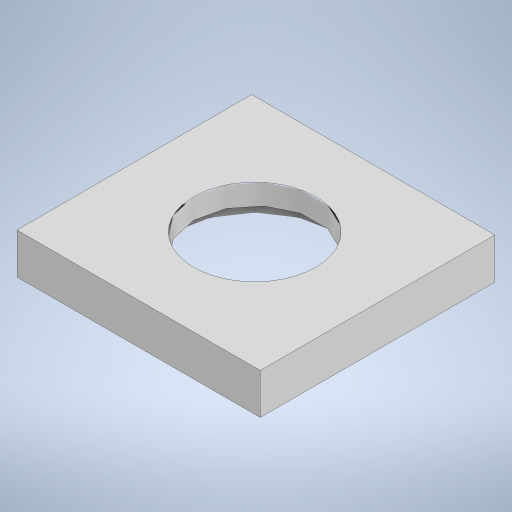
# Autodesk Inventor part: Button_slot
Saved by Autodesk Inventor 2023 (Build 270158000, 158)
## iProperties
Created: 2022-11-29
Part Number: Button_slot
Material: Generic
Document SubType Name: Modeling
Designer: spfow
Density: 1 g/cm^3
Appearance: Default
Author: spfow
Autodesk Inventor part; units mm, degrees
note: some values were not read from the file. Chosen so that the rebuilt part matches the saved one: offset side.
ref_plane "YZ Plane" through (0, 0, 0) normal (1, 0, 0) x (0, 1, 0)
ref_plane "XZ Plane" through (0, 0, 0) normal (0, 1, 0) x (-1, 0, 0)
ref_plane "XY Plane" through (0, 0, 0) normal (0, 0, 1) x (1, 0, 0)
sketch "Sketch1" plane through (0, 0, 0) normal (0, 1, 0) x (-1, 0, 0)
  line L0 (0, 0) -> (177.8, 0)
  line L1 (177.8, 0) -> (177.8, -114.3)
  line L2 (177.8, -114.3) -> (0, -114.3)
  line L3 (0, -114.3) -> (0, 0)
  dimension "d0" = 177.8
  dimension "d1" = 114.3
  constraints: 8 end point, 2 parallel, 1 horizontal, 1 perpendicular
  measures "d0" distance of L1.end L2.end
  measures "d1" distance of L0.end L1.end
extrude "Extrusion1" add sketch "Sketch1" along normal blind 38.1
sketch "Sketch2" plane through (0, 0, 0) normal (0, -1, 0) x (1, 0, 0)
  line L0 (-177.8, -114.3) -> (-177.8, 0) projected
  line L1 (0, 0) -> (-177.8, 0)
  line L2 (-177.8, 0) -> (-177.8, -114.3)
  line L3 (-177.8, -114.3) -> (0, -114.3)
  line L4 (0, -114.3) -> (0, 0)
  line L5 (-5.08, -5.08) -> (-172.72, -5.08)
  line L6 (-172.72, -5.08) -> (-172.72, -109.22)
  line L7 (-172.72, -109.22) -> (-5.08, -109.22)
  line L8 (-5.08, -109.22) -> (-5.08, -5.08)
  dimension "d4" = 5.08
  constraints: 16 end point, 4 parallel, 2 perpendicular, 1 horizontal, 3 other
  measures "d4" distance between parallel lines of L4 L8
extrude "Extrusion2" cut sketch "Sketch2" against normal blind 35.56 contours L8 L7 L6 L5
fillet "Fillet1" radius 3.175 4 edges at (-177.8, 38.1, -57.15) (-88.9, 38.1, 0) (-88.9, 38.1, -114.3) (0, 38.1, -57.15)
sketch "Sketch3" plane through (0, 38.1, 0) normal (0, 1, 0) x (1, 0, 0)
  line L0 (-177.8, 114.3) -> (-171.45, 114.3)
  line L1 (-171.45, 114.3) -> (-171.45, 0)
  line L2 (-171.45, 0) -> (-177.8, 0)
  line L3 (-177.8, 0) -> (-177.8, 114.3)
  line L4 (0, 114.3) -> (-177.8, 114.3) projected
  line L5 (-177.8, 114.3) -> (0, 114.3)
  line L6 (0, 114.3) -> (0, 107.95)
  line L7 (0, 107.95) -> (-177.8, 107.95)
  line L8 (-177.8, 107.95) -> (-177.8, 114.3)
  line L9 (-158.75, 100.4887) -> (-100.6475, 100.4887)
  line L10 (-100.6475, 100.4887) -> (-100.6475, 13.8112)
  line L11 (-100.6475, 13.8112) -> (-158.75, 13.8112)
  line L12 (-158.75, 13.8112) -> (-158.75, 100.4887)
  point P0 (0, 0)
  dimension "d8" = 6.35
  dimension "d9" = 6.35
  dimension "d10" = 58.1025
  dimension "d11" = 86.6775
  dimension "d12" = 13.8112
  dimension "d13" = 19.05
  constraints: 24 end point, 6 parallel, 3 horizontal, 3 perpendicular
  measures "d8" distance of L1.end L2.end
  measures "d9" distance of L5.end L6.end
  measures "d10" distance of L9.start L9.end
  measures "d11" distance of L9.end L10.end
  measures "d12" distance between parallel lines of L4 L9
  measures "d13" distance between parallel lines of L3 L12
extrude "Extrusion3" cut sketch "Sketch3" against normal blind 35.56 contours L9 L10 L11 L12
sketch "Sketch4" plane through (0, 38.1, 0) normal (0, 1, 0) x (1, 0, 0)
  line L0 (-94.2975, 17.78) -> (-81.2088, 17.78)
  line L1 (-91.7575, 20.32) -> (-91.7575, 26.67)
  line L2 (-91.7575, 26.67) -> (-94.2975, 26.67)
  line L3 (-94.2975, 26.67) -> (-94.2975, 17.78)
  line L4 (-94.2975, 17.78) -> (-78.6765, 17.78)
  line L5 (-78.6765, 17.78) -> (-78.6765, 20.32)
  line L6 (-94.2975, 24.2647) -> (-94.2975, 17.78)
  line L7 (-85.6615, 20.32) -> (-85.6615, 24.13)
  line L8 (-85.6615, 24.13) -> (-88.2015, 24.13)
  line L9 (-88.2015, 24.13) -> (-88.2015, 20.32)
  line L10 (-78.6765, 20.32) -> (-85.6615, 20.32)
  line L11 (-88.2015, 20.32) -> (-91.7575, 20.32)
  line L12 (-100.6475, 100.4887) -> (-100.6475, 13.8112) projected
  line L13 (-177.8, 0) -> (0, 0) projected
  line L14 (-94.2975, 27.94) -> (-78.6765, 27.94)
  line L15 (-78.6765, 27.94) -> (-78.6765, 30.7699)
  line L16 (-81.2165, 30.48) -> (-94.2975, 30.48)
  line L17 (-94.2975, 30.48) -> (-94.2975, 27.94)
  line L18 (-83.0828, 27.94) -> (-78.6765, 27.94)
  line L19 (-78.6765, 27.94) -> (-78.6765, 36.83)
  line L20 (-78.6765, 36.83) -> (-81.2165, 36.83)
  line L21 (-81.2165, 36.83) -> (-81.2165, 30.48)
  ellipse E0 centre (-86.487, 41.91) end of major axis (-94.2975, 41.91) minor radius 5.334
  ellipse E1 centre (-86.487, 53.34) end of major axis (-94.2975, 53.34) minor radius 5.334
  line L22 (-94.2975, 60.96) -> (-78.6765, 60.96)
  line L23 (-78.6765, 60.96) -> (-78.6765, 63.754)
  line L24 (-94.2975, 63.754) -> (-94.2975, 60.96)
  ellipse E2 centre (-86.487, 63.754) end of major axis (-94.2975, 63.754) minor radius 7.62 (-78.6765, 63.754) -> (-94.2975, 63.754) ccw
  line L25 (-91.7575, 63.754) -> (-91.7575, 63.5)
  line L26 (-91.7575, 63.5) -> (-81.2165, 63.5)
  line L27 (-81.2165, 63.5) -> (-81.2165, 63.754)
  line L28 (-94.2975, 82.55) -> (-78.6765, 82.55)
  line L29 (-78.6765, 82.55) -> (-78.6765, 80.01)
  line L30 (-78.6765, 80.01) -> (-94.2975, 80.01)
  line L31 (-94.2975, 80.01) -> (-94.2975, 82.55)
  line L32 (-91.7575, 89.535) -> (-78.6765, 89.535)
  line L33 (-78.6765, 89.535) -> (-78.6765, 92.075)
  line L34 (-78.6765, 92.075) -> (-91.7575, 92.075)
  line L35 (-94.2975, 94.8241) -> (-94.2975, 91.9305)
  line L36 (-94.2975, 85.09) -> (-91.7575, 85.09)
  line L37 (-91.7575, 96.52) -> (-94.2975, 96.52)
  line L38 (-94.2975, 96.52) -> (-94.2975, 85.09)
  line L39 (-91.7575, 85.09) -> (-91.7575, 89.535)
  line L40 (-91.7575, 92.075) -> (-91.7575, 96.52)
  spline S0 degree 5 poles (-91.7575, 41.91) (-91.7584, 41.6813) (-91.6944, 41.4527) (-91.5885, 41.2473) (-91.2042, 40.6846) (-90.6636, 40.2564) (-90.282, 40.0177) (-89.3306, 39.5478) (-88.3046, 39.2718) (-87.7026, 39.1679) (-86.487, 39.0641) (-85.2714, 39.1679) (-84.6694, 39.2718) (-83.6435, 39.5478) (-82.692, 40.0176) (-82.3107, 40.2563) (-81.7696, 40.6845) (-81.3858, 41.2473) (-81.2787, 41.4526) (-81.1539, 41.91) (-81.2787, 42.3674) (-81.3858, 42.5727) (-81.7696, 43.1355) (-82.3107, 43.5637) (-82.692, 43.8024) (-83.6435, 44.2722) (-84.6694, 44.5482) (-85.2714, 44.6521) (-86.487, 44.7559) (-87.7026, 44.6521) (-88.3046, 44.5482) (-89.3306, 44.2722) (-90.282, 43.8023) (-90.6636, 43.5636) (-91.2042, 43.1354) (-91.5885, 42.5727) (-91.6944, 42.3673) (-91.7584, 42.1387) (-91.7575, 41.91) knots 0 0 0 0 0 0 0.044471 0.044471 0.044471 0.131758 0.131758 0.131758 0.25 0.25 0.25 0.36824 0.36824 0.36824 0.455522 0.455522 0.455522 0.5 0.5 0.5 0.544478 0.544478 0.544478 0.63176 0.63176 0.63176 0.75 0.75 0.75 0.868242 0.868242 0.868242 0.955529 0.955529 0.955529 1 1 1 1 1 1
  spline S1 degree 5 poles (-91.7575, 53.34) (-91.7584, 53.1113) (-91.6944, 52.8827) (-91.5885, 52.6773) (-91.2042, 52.1146) (-90.6636, 51.6864) (-90.282, 51.4477) (-89.3306, 50.9778) (-88.3046, 50.7018) (-87.7026, 50.5979) (-86.487, 50.4941) (-85.2714, 50.5979) (-84.6694, 50.7018) (-83.6435, 50.9778) (-82.692, 51.4476) (-82.3107, 51.6863) (-81.7696, 52.1145) (-81.3858, 52.6773) (-81.2787, 52.8826) (-81.1539, 53.34) (-81.2787, 53.7974) (-81.3858, 54.0027) (-81.7696, 54.5655) (-82.3107, 54.9937) (-82.692, 55.2324) (-83.6435, 55.7022) (-84.6694, 55.9782) (-85.2714, 56.0821) (-86.487, 56.1859) (-87.7026, 56.0821) (-88.3046, 55.9782) (-89.3306, 55.7022) (-90.282, 55.2323) (-90.6636, 54.9936) (-91.2042, 54.5654) (-91.5885, 54.0027) (-91.6944, 53.7973) (-91.7584, 53.5687) (-91.7575, 53.34) knots 0 0 0 0 0 0 0.044471 0.044471 0.044471 0.131758 0.131758 0.131758 0.25 0.25 0.25 0.36824 0.36824 0.36824 0.455522 0.455522 0.455522 0.5 0.5 0.5 0.544478 0.544478 0.544478 0.63176 0.63176 0.63176 0.75 0.75 0.75 0.868242 0.868242 0.868242 0.955529 0.955529 0.955529 1 1 1 1 1 1
  spline S2 degree 5 poles (-81.2165, 63.754) (-81.2166, 64.309) (-81.2953, 64.8639) (-81.4525, 65.404) (-82.1282, 66.8995) (-83.3585, 68.0474) (-84.3453, 68.5716) (-86.487, 69.0964) (-88.6287, 68.5716) (-89.6155, 68.0474) (-90.8458, 66.8995) (-91.5215, 65.404) (-91.6787, 64.8639) (-91.7574, 64.309) (-91.7575, 63.754) knots 0 0 0 0 0 0 0.170659 0.170659 0.170659 0.5 0.5 0.5 0.829341 0.829341 0.829341 1 1 1 1 1 1
  point P0 (-94.2975, 93.3773)
  point P1 (-88.9, 0)
  point P2 (-93.0275, 85.09)
  dimension "d32" = 5.334
  dimension "d33" = 7.8105
  dimension "d36" = 7.8105
  dimension "d37" = 5.334
  dimension "d42" = 7.62
  dimension "d43" = 2.54
  dimension "d16" = 2.54
  dimension "d17" = 3.556
  dimension "d18" = 2.54
  dimension "d19" = 6.985
  dimension "d20" = 8.89
  dimension "d21" = 6.35
  dimension "d22" = 3.81
  dimension "d23" = 3.81
  dimension "d24" = 6.35
  dimension "d25" = 17.78
  dimension "d26" = 2.54
  dimension "d27" = 2.54
  dimension "d28" = 6.35
  dimension "d29" = 15.621
  dimension "d30" = 6.35
  dimension "d31" = 27.94
  dimension "d34" = 14.1605
  dimension "d35" = 41.91
  dimension "d38" = 14.1605
  dimension "d39" = 53.34
  dimension "d40" = 2.54
  dimension "d41" = 2.54
  dimension "d44" = 6.35
  dimension "d45" = 15.621
  dimension "d46" = 60.96
  dimension "d47" = 2.794
  dimension "d48" = 63.754
  dimension "d49" = 14.1605
  dimension "d50" = 2.54
  dimension "d51" = 15.621
  dimension "d52" = 4.445
  dimension "d53" = 4.445
  dimension "d54" = 2.54
  dimension "d55" = 2.54
  dimension "d56" = 6.35
  dimension "d57" = 80.01
  dimension "d58" = 2.54
  dimension "d59" = 13.081
  dimension "d62" = 3.9688
  dimension "d63" = 3.9688
  constraints: 78 end point, 20 parallel, 10 perpendicular, 8 horizontal, 5 point on line, 3 midpoint, 13 other
  measures "d16" distance of L1.end L2.end
  measures "d17" distance of L9.end L1.start
  measures "d18" distance of L7.end L8.end
  measures "d19" distance of L5.end L7.start
  measures "d20" distance of L2.end L0.start
  measures "d21" distance of L1.start L1.end
  measures "d22" distance of L8.end L9.end
  measures "d23" distance of L7.start L7.end
  measures "d24" distance between parallel lines of L12 L3
  measures "d25" distance between parallel lines of L13 L0
  measures "d26" distance of L16.end L14.start
  measures "d27" distance of L19.end L20.end
  measures "d28" distance of L20.end L16.start
  measures "d29" distance of L14.start L14.end
  measures "d30" distance between parallel lines of L12 L17
  measures "d31" distance between parallel lines of L13 L14
  measures "d34" distance from line of L12 point (-86.487, 41.91)
  measures "d35" distance from line of L13 point (-86.487, 41.91)
  measures "d38" distance from line of L12 point (-86.487, 53.34)
  measures "d39" distance from line of L13 point (-86.487, 53.34)
  measures "d44" distance between parallel lines of L12 L24
  measures "d45" distance of L22.start L22.end
  measures "d46" distance between parallel lines of L13 L22
  measures "d47" distance of L24.start L22.start
  measures "d48" distance from line of L13 point (-86.487, 63.754)
  measures "d49" distance from line of L12 point (-86.487, 63.754)
  measures "d50" distance of L30.end L28.start
  measures "d51" distance of L29.end L30.end
  measures "d52" distance of L36.end L32.start
  measures "d53" distance of L34.end L37.start
  measures "d54" distance between parallel lines of L32 L34
  measures "d55" distance between parallel lines of L40 L38
  measures "d56" distance from line of L12 point (-94.298, 93.377)
  measures "d57" distance from line of point (-88.9, 0) L30
  measures "d58" distance from line of L28 point (-93.028, 85.09)
  measures "d59" distance of L32.start L32.end
  measures "d62" distance from line of L12.start L37
  measures "d63" distance from line of L12.end L0
extrude "Extrusion4" cut sketch "Sketch4" against normal blind 1.27
sketch "Sketch5" plane through (0, 38.1, 0) normal (0, 1, 0) x (1, 0, 0)
  line L0 (-43.4975, 22.6219) -> (-37.9413, 22.6219)
  line L1 (-37.9413, 22.6219) -> (-37.9413, 28.1781)
  line L2 (-37.9413, 28.1781) -> (-43.4975, 28.1781)
  line L3 (-43.4975, 28.1781) -> (-43.4975, 22.6219)
  line L4 (-43.4975, 38.4969) -> (-37.9413, 38.4969)
  line L5 (-37.9413, 38.4969) -> (-37.9413, 44.0531)
  line L6 (-37.9413, 44.0531) -> (-43.4975, 44.0531)
  line L7 (-43.4975, 44.0531) -> (-43.4975, 38.4969)
  line L8 (-43.4975, 54.3719) -> (-37.9413, 54.3719)
  line L9 (-37.9413, 54.3719) -> (-37.9413, 59.9281)
  line L10 (-37.9413, 59.9281) -> (-43.4975, 59.9281)
  line L11 (-43.4975, 59.9281) -> (-43.4975, 54.3719)
  line L12 (-43.4975, 70.2469) -> (-37.9413, 70.2469)
  line L13 (-37.9413, 70.2469) -> (-37.9413, 75.8031)
  line L14 (-37.9413, 75.8031) -> (-43.4975, 75.8031)
  line L15 (-43.4975, 75.8031) -> (-43.4975, 70.2469)
  line L16 (-43.4975, 86.1219) -> (-37.9413, 86.1219)
  line L17 (-37.9413, 86.1219) -> (-37.9413, 91.6781)
  line L18 (-37.9413, 91.6781) -> (-43.4975, 91.6781)
  line L19 (-43.4975, 91.6781) -> (-43.4975, 86.1219)
  line L20 (0, 114.3) -> (-177.8, 114.3) projected
  line L21 (-177.8, 0) -> (0, 0) projected
  line L22 (-100.6475, 100.4887) -> (-100.6475, 13.8112) projected
  circle A0 centre (-21.9075, 25.4) radius 3.81
  circle A1 centre (-21.9075, 41.275) radius 3.81
  circle A2 centre (-21.9075, 57.15) radius 3.81
  circle A3 centre (-21.9075, 73.025) radius 3.81
  circle A4 centre (-21.9075, 88.9) radius 3.81
  point P0 (-43.4975, 73.025)
  dimension "d64" = 5.5563
  dimension "d65" = 5.5563
  dimension "d66" = 5.5563
  dimension "d67" = 5.5563
  dimension "d68" = 5.5563
  dimension "d69" = 5.5563
  dimension "d70" = 15.875
  dimension "d71" = 15.875
  dimension "d72" = 15.875
  dimension "d73" = 15.875
  dimension "d74" = 22.6219
  dimension "d76" = 57.15
  dimension "d77" = 7.62
  dimension "d78" = 7.62
  dimension "d79" = 7.62
  dimension "d80" = 7.62
  dimension "d81" = 7.62
  dimension "d82" = 15.875
  dimension "d83" = 15.875
  dimension "d84" = 15.875
  dimension "d85" = 15.875
  dimension "d86" = 25.4
  dimension "d87" = 78.74
  dimension "d88" = 78.74
  dimension "d89" = 78.74
  dimension "d90" = 78.74
  dimension "d91" = 78.74
  constraints: 40 end point, 10 parallel, 8 point on line, 5 centre point, 5 horizontal, 5 perpendicular, 1 midpoint
  measures "d64" distance of L2.end L0.start
  measures "d65" distance of L6.end L4.start
  measures "d66" distance of L10.end L8.start
  measures "d67" distance of L14.end L12.start
  measures "d68" distance of L18.end L16.start
  measures "d69" distance of L17.end L18.end
  measures "d70" distance of L5.end L1.end
  measures "d71" distance of L9.end L5.end
  measures "d72" distance of L13.end L9.end
  measures "d73" distance of L17.end L13.end
  measures "d74" distance between parallel lines of L20 L18
  measures "d76" distance from line of point (-43.498, 73.025) L22
  measures "d77" diameter of A0
  measures "d78" diameter of A1
  measures "d79" diameter of A2
  measures "d80" diameter of A3
  measures "d81" diameter of A4
  measures "d82" distance of A1.centre A0.centre
  measures "d83" distance of A2.centre A1.centre
  measures "d84" distance of A3.centre A2.centre
  measures "d85" distance of A4.centre A3.centre
  measures "d86" distance from line of L20 A4.centre
  measures "d87" distance from line of L22 A2.centre
  measures "d88" distance from line of L22 A3.centre
  measures "d89" distance from line of L22 A4.centre
  measures "d90" distance from line of L22 A1.centre
  measures "d91" distance from line of L22 A0.centre
extrude "Extrusion5" cut sketch "Sketch5" against normal blind 25.4
sketch "Sketch6" plane through (0, 35.56, 0) normal (0, -1, 0) x (1, 0, 0)
  circle A0 centre (-21.9075, -88.9) radius 3.81 projected
  circle A1 centre (-21.9075, -88.9) radius 5.08
  circle A2 centre (-21.9075, -73.025) radius 3.81 projected
  circle A3 centre (-21.9075, -73.025) radius 5.08
  circle A4 centre (-21.9075, -57.15) radius 3.81 projected
  circle A5 centre (-21.9075, -57.15) radius 5.08
  circle A6 centre (-21.9075, -41.275) radius 3.81 projected
  circle A7 centre (-21.9075, -41.275) radius 5.08
  circle A8 centre (-21.9075, -25.4) radius 3.81 projected
  circle A9 centre (-21.9075, -25.4) radius 5.08
  line L0 (-43.4975, -59.9281) -> (-37.9413, -59.9281)
  line L1 (-37.9413, -59.9281) -> (-37.9413, -54.3719)
  line L2 (-37.9413, -54.3719) -> (-43.4975, -54.3719)
  line L3 (-43.4975, -54.3719) -> (-43.4975, -59.9281)
  line L4 (-45.4025, -61.8331) -> (-36.0363, -61.8331)
  line L5 (-36.0363, -61.8331) -> (-36.0363, -52.4669)
  line L6 (-36.0363, -52.4669) -> (-45.4025, -52.4669)
  line L7 (-45.4025, -52.4669) -> (-45.4025, -61.8331)
  line L8 (-43.4975, -91.6781) -> (-37.9413, -91.6781)
  line L9 (-37.9413, -91.6781) -> (-37.9413, -86.1219)
  line L10 (-37.9413, -86.1219) -> (-43.4975, -86.1219)
  line L11 (-43.4975, -86.1219) -> (-43.4975, -91.6781)
  line L12 (-43.4975, -75.8031) -> (-37.9413, -75.8031) projected
  line L13 (-37.9413, -70.2469) -> (-36.6713, -68.9769) projected
  line L14 (-43.4975, -75.8031) -> (-37.9413, -75.8031)
  line L15 (-37.9413, -75.8031) -> (-37.9413, -70.2469)
  line L16 (-37.9413, -70.2469) -> (-43.4975, -70.2469)
  line L17 (-43.4975, -70.2469) -> (-43.4975, -75.8031)
  line L18 (-43.4975, -38.4969) -> (-43.4975, -44.0531) projected
  line L19 (-43.4975, -44.0531) -> (-37.9413, -44.0531)
  line L20 (-37.9413, -44.0531) -> (-37.9413, -38.4969)
  line L21 (-37.9413, -38.4969) -> (-43.4975, -38.4969)
  line L22 (-43.4975, -38.4969) -> (-43.4975, -44.0531)
  line L23 (-37.9413, -28.1781) -> (-43.4975, -28.1781) projected
  line L24 (-37.9413, -22.6219) -> (-36.6713, -21.3519) projected
  line L25 (-43.4975, -28.1781) -> (-37.9413, -28.1781)
  line L26 (-37.9413, -28.1781) -> (-37.9413, -22.6219)
  line L27 (-37.9413, -22.6219) -> (-43.4975, -22.6219)
  line L28 (-43.4975, -22.6219) -> (-43.4975, -28.1781)
  line L29 (-45.4025, -77.7081) -> (-36.0363, -77.7081)
  line L30 (-36.0363, -77.7081) -> (-36.0363, -68.3419)
  line L31 (-36.0363, -68.3419) -> (-45.4025, -68.3419)
  line L32 (-45.4025, -68.3419) -> (-45.4025, -77.7081)
  line L33 (-45.4025, -84.2169) -> (-36.0362, -84.2169)
  line L34 (-36.0362, -84.2169) -> (-36.0362, -93.5831)
  line L35 (-36.0362, -93.5831) -> (-45.4025, -93.5831)
  line L36 (-45.4025, -93.5831) -> (-45.4025, -84.2169)
  line L37 (-36.0362, -45.9581) -> (-45.4025, -45.9581)
  line L38 (-45.4025, -45.9581) -> (-45.4025, -36.5919)
  line L39 (-45.4025, -36.5919) -> (-36.0362, -36.5919)
  line L40 (-36.0362, -36.5919) -> (-36.0362, -45.9581)
  line L41 (-45.4025, -30.0831) -> (-36.0363, -30.0831)
  line L42 (-36.0363, -30.0831) -> (-36.0363, -20.7169)
  line L43 (-36.0363, -20.7169) -> (-45.4025, -20.7169)
  line L44 (-45.4025, -20.7169) -> (-45.4025, -30.0831)
  line L45 (-48.3394, -99.6918) -> (-33.0994, -99.6918)
  line L46 (-33.0994, -99.6918) -> (-33.0994, -14.6018)
  line L47 (-33.0994, -14.6018) -> (-48.3394, -14.6018)
  line L48 (-48.3394, -14.6018) -> (-48.3394, -99.6918)
  point P0 (0, 0)
  point P1 (-43.4975, -38.4969)
  point P2 (-40.7194, -44.0531)
  point P3 (-40.7194, -91.6781)
  point P4 (-40.7194, -14.6018)
  dimension "d97" = 10.16
  dimension "d98" = 10.16
  dimension "d99" = 10.16
  dimension "d100" = 10.16
  dimension "d101" = 10.16
  dimension "d119" = 1.905
  dimension "d120" = 1.905
  dimension "d121" = 1.905
  dimension "d122" = 1.905
  dimension "d123" = 1.905
  dimension "d136" = 15.24
  dimension "d137" = 85.09
  dimension "d139" = 7.62
  dimension "d140" = 8.0137
  dimension "d141" = 8.02
  constraints: 88 end point, 22 parallel, 11 perpendicular, 6 horizontal, 5 centre point, 5 coincident, 3 midpoint, 15 other
  measures "d97" diameter of A1
  measures "d98" diameter of A3
  measures "d99" diameter of A5
  measures "d100" diameter of A7
  measures "d101" diameter of A9
  measures "d119" distance between parallel lines of L3 L7
  measures "d120" distance between parallel lines of L17 L32
  measures "d121" distance between parallel lines of L10 L33
  measures "d122" distance between parallel lines of L19 L37
  measures "d123" distance between parallel lines of L28 L44
  measures "d136" distance of L45.start L45.end
  measures "d137" distance of L47.end L45.start
  measures "d139" distance from line of point (-40.719, -44.053) L48
  measures "d140" distance from line of L45 point (-40.719, -91.678)
  measures "d141" distance from line of point (-40.719, -14.602) L27
extrude "Extrusion6" cut sketch "Sketch6" against normal blind 1.27 contours A1 | A3 | A5 | A7 | A9
extrude "Extrusion9" cut sketch "Sketch6" against normal blind 1.7463 contours L7 L6 L5 L4 | L32 L31 L30 L29 | L33 L34 L35 L36 | L37 L38 L39 L40 | L44 L43 L42 L41
sketch "Sketch8" plane through (0, 35.56, 0) normal (0, -1, 0) x (1, 0, 0)
  line L0 (-100.6475, -13.8112) -> (-100.6475, -100.4887) projected
  line L1 (-100.6475, -13.8112) -> (-158.75, -13.8112)
  line L2 (-158.75, -13.8112) -> (-158.75, -7.4613)
  line L3 (-158.75, -7.4613) -> (-100.6475, -7.4612)
  line L4 (-100.6475, -7.4612) -> (-100.6475, -13.8112)
  line L5 (-158.75, -100.4887) -> (-100.6475, -100.4887) projected
  line L6 (-100.6475, -100.4887) -> (-158.75, -100.4887)
  line L7 (-158.75, -100.4887) -> (-158.75, -107.4737)
  line L8 (-158.75, -107.4737) -> (-100.6475, -107.4737)
  line L9 (-100.6475, -107.4737) -> (-100.6475, -100.4887)
  line L10 (-100.6475, -7.4612) -> (-94.2975, -7.4612)
  line L11 (-94.2975, -7.4612) -> (-94.2975, -13.8112)
  line L12 (-94.2975, -13.8112) -> (-100.6475, -13.8112)
  line L13 (-100.6475, -13.8112) -> (-100.6475, -7.4612)
  line L14 (-100.6475, -100.4887) -> (-94.2975, -100.4887)
  line L15 (-94.2975, -100.4887) -> (-94.2975, -107.4737)
  line L16 (-94.2975, -107.4737) -> (-100.6475, -107.4737)
  line L17 (-100.6475, -107.4737) -> (-100.6475, -100.4887)
  line L18 (-158.75, -100.4887) -> (-165.1, -100.4887)
  line L19 (-165.1, -100.4887) -> (-165.1, -107.4737)
  line L20 (-165.1, -107.4737) -> (-158.75, -107.4737)
  line L21 (-158.75, -107.4737) -> (-158.75, -100.4887)
  line L22 (-158.75, -7.4613) -> (-165.1, -7.4613)
  line L23 (-165.1, -7.4613) -> (-165.1, -13.8112)
  line L24 (-165.1, -13.8112) -> (-158.75, -13.8112)
  line L25 (-158.75, -13.8112) -> (-158.75, -7.4613)
  line L26 (-102.4053, -9.0487) -> (-155.7453, -9.0487)
  line L27 (-155.7453, -9.0487) -> (-155.7453, -12.2237)
  line L28 (-155.7453, -12.2237) -> (-102.4053, -12.2237)
  line L29 (-102.4053, -12.2237) -> (-102.4053, -9.0487)
  point P0 (0, 0)
  dimension "d126" = 6.35
  dimension "d127" = 6.985
  dimension "d128" = 6.35
  dimension "d129" = 6.35
  dimension "d130" = 6.35
  dimension "d131" = 53.34
  dimension "d132" = 3.175
  dimension "d133" = 1.5875
  constraints: 56 end point, 14 parallel, 7 horizontal, 7 perpendicular, 2 point on line
  measures "d126" distance of L3.end L0.start
  measures "d127" distance of L8.end L0.end
  measures "d128" distance of L11.end L12.end
  measures "d129" distance of L20.end L19.end
  measures "d130" distance of L24.end L23.end
  measures "d131" distance of L28.end L27.end
  measures "d132" distance between parallel lines of L28 L26
  measures "d133" distance between parallel lines of L1 L28
extrude "Extrusion10" cut sketch "Sketch8" against normal blind 1.27 contours L29 L28 L27 L26
extrude "Extrusion11" cut sketch "Sketch6" against normal blind 0.9525 contours L48 L47 L46 L45
sketch "Sketch9" plane through (-177.8, 0, 0) normal (0, 0, 1) x (1, 0, 0)
  line L0 (77.1525, 35.56) -> (19.05, 35.56) projected
  line L1 (172.72, 0) -> (5.08, 0) projected
  line L2 (77.1525, 35.56) -> (127.9525, 35.56)
  line L3 (127.9525, 35.56) -> (127.9525, 0)
  line L4 (127.9525, 0) -> (77.1525, 0)
  line L5 (77.1525, 0) -> (77.1525, 35.56)
  line L6 (86.0425, 17.145) -> (106.68, 17.145)
  line L7 (106.68, 17.145) -> (106.68, 15.0495)
  line L8 (106.68, 15.0495) -> (86.0425, 15.0495)
  line L9 (86.0425, 15.0495) -> (86.0425, 17.145)
  line L10 (88.5825, 15.0495) -> (97.4725, 15.0495)
  line L11 (97.4725, 15.0495) -> (97.4725, 11.2395)
  line L12 (97.4725, 11.2395) -> (88.5825, 11.2395)
  line L13 (88.5825, 11.2395) -> (88.5825, 15.0495)
  line L14 (0, 34.925) -> (177.8, 34.925) projected
  line L15 (0, 0) -> (0, 34.925) projected
  line L16 (177.8, 0) -> (177.8, 34.925) projected
  point P0 (97.4725, 15.0495)
  dimension "d144" = 50.8
  dimension "d145" = 20.6375
  dimension "d146" = 2.0955
  dimension "d147" = 8.89
  dimension "d148" = 3.81
  dimension "d149" = 2.54
  dimension "d150" = 17.78
  dimension "d187" = 71.12
  constraints: 24 end point, 6 parallel, 3 horizontal, 3 perpendicular, 2 point on line
  measures "d144" distance of L3.end L4.end
  measures "d145" distance of L6.start L6.end
  measures "d146" distance of L6.end L7.end
  measures "d147" distance of L11.end L12.end
  measures "d148" distance of L10.end L11.end
  measures "d149" distance between parallel lines of L9 L13
  measures "d150" distance between parallel lines of L14 L6
  measures "d187" distance between parallel lines of L16 L7
extrude "Extrusion12" cut sketch "Sketch9" against normal blind 5.08 contours L6 L7 L8 L9 | L8 L11 L12 L13
sketch "Sketch10" plane through (-5.08, 0, -5.08) normal (0, 0, -1) x (-1, 0, 0)
  line L0 (84.1375, 11.2395) -> (75.2475, 11.2395) projected
  line L1 (84.1375, 15.0495) -> (86.6775, 15.0495) projected
  line L2 (75.2475, 11.2395) -> (84.1375, 11.2395)
  line L3 (84.1375, 11.2395) -> (84.1375, 15.0495)
  line L4 (75.2475, 15.0495) -> (75.2475, 11.2395)
  line L5 (75.2475, 15.0495) -> (66.04, 15.0495) projected
  line L6 (86.6775, 17.145) -> (86.6775, 15.0495) projected
  line L7 (86.6775, 15.0495) -> (86.6775, 17.145)
  line L8 (86.6775, 17.145) -> (66.04, 17.145)
  line L9 (66.04, 17.145) -> (66.04, 15.0495)
  line L10 (66.04, 15.0495) -> (75.2475, 15.0495)
  line L11 (84.1375, 15.0495) -> (86.6775, 15.0495)
  line L12 (73.3425, 9.3345) -> (86.0425, 9.3345)
  line L13 (86.0425, 9.3345) -> (86.0425, 13.1445)
  line L14 (86.0425, 13.1445) -> (88.5825, 13.1445)
  line L15 (88.5825, 13.1445) -> (88.5825, 19.05)
  line L16 (88.5825, 19.05) -> (64.135, 19.05)
  line L17 (64.135, 19.05) -> (64.135, 13.1445)
  line L18 (64.135, 13.1445) -> (73.3425, 13.1445)
  line L19 (73.3425, 13.1445) -> (73.3425, 9.3345)
  line L20 (73.3425, 13.1445) -> (73.3425, 15.0495)
  line L21 (86.0425, 13.1445) -> (86.0425, 15.0495)
  point P0 (-5.08, 0)
  dimension "d153" = 1.905
  constraints: 36 end point, 9 parallel, 7 perpendicular, 3 horizontal, 2 point on line, 7 other
  measures "d153" distance between parallel lines of L4 L19
extrude "Extrusion13" cut sketch "Sketch10" against normal blind 3.175 contours L3 L1 L21 L13 L12 L19 L20 L5 L4 L0 | L1 L6 L8 L9 L5 L20 L18 L17 L16 L15 L14 L21
sketch "Sketch11" plane through (0, 0, -114.3) normal (0, 0, -1) x (-1, 0, 0)
  line L0 (63.5, 23.495) -> (76.2, 23.495)
  line L1 (76.2, 23.495) -> (76.2, 15.875)
  line L2 (76.2, 15.875) -> (63.5, 15.875)
  line L3 (63.5, 15.875) -> (63.5, 23.495)
  line L4 (0, 0) -> (0, 34.925) projected
  circle A0 centre (69.85, 19.685) radius 3.81
  line L5 (0, 34.925) -> (177.8, 34.925) projected
  dimension "d156" = 7.62
  dimension "d157" = 63.5
  dimension "d158" = 12.7
  dimension "d164" = 11.43
  dimension "d165" = 15.24
  constraints: 8 end point, 2 parallel, 1 centre point, 1 horizontal, 1 perpendicular
  measures "d156" distance of L0.end L1.end
  measures "d157" distance between parallel lines of L4 L3
  measures "d158" distance of L0.start L0.end
  measures "d164" distance between parallel lines of L5 L0
  measures "d165" distance from line of L5 A0.centre
extrude "Extrusion14" cut sketch "Sketch11" against normal blind 6.35 contours A0
sketch "Sketch12" plane through (-172.72, 0, -109.22) normal (0, 0, 1) x (1, 0, 0)
  line L0 (96.52, 15.875) -> (109.22, 15.875)
  line L1 (109.22, 15.875) -> (109.22, 23.495)
  line L2 (109.22, 23.495) -> (96.52, 23.495)
  line L3 (96.52, 23.495) -> (96.52, 15.875)
  circle A0 centre (102.87, 19.685) radius 3.81 projected
  line L4 (96.52, 15.875) -> (109.22, 23.495) construction
  line L5 (109.22, 15.875) -> (96.52, 23.495) construction
  point P0 (172.72, 0)
  point P1 (102.87, 15.875)
  point P2 (102.87, 23.495)
  dimension "d161" = 12.7
  constraints: 12 end point, 2 midpoint, 2 parallel, 1 horizontal, 1 perpendicular
  measures "d161" distance of L0.start L0.end
extrude "Extrusion15" cut sketch "Sketch12" against normal blind 2.0574 contours L3 L2 A0 L0 | A0 L2 L1 L0
sketch "Sketch13" plane through (0, 35.56, 0) normal (0, -1, 0) x (1, 0, 0)
  line L0 (-48.3394, -99.6918) -> (-48.3394, -14.6018) projected
  line L1 (-48.3394, -31.1933) -> (-46.4344, -31.1933)
  line L2 (-46.4344, -31.1933) -> (-46.4344, -36.2733)
  line L3 (-46.4344, -36.2733) -> (-48.3394, -36.2733)
  line L4 (-48.3394, -36.2733) -> (-48.3394, -31.1933)
  line L5 (-33.0994, -14.6018) -> (-33.0994, -99.6918) projected
  line L6 (-33.0994, -36.2733) -> (-35.0044, -36.2733)
  line L7 (-35.0044, -36.2733) -> (-35.0044, -31.1933)
  line L8 (-35.0044, -31.1933) -> (-33.0994, -31.1933)
  line L9 (-33.0994, -31.1933) -> (-33.0994, -36.2733)
  line L10 (-46.4344, -31.1933) -> (-51.5144, -31.1933)
  line L11 (-51.5144, -31.1933) -> (-51.5144, -36.2733)
  line L12 (-51.5144, -36.2733) -> (-46.4344, -36.2733)
  line L13 (-46.4344, -36.2733) -> (-46.4344, -31.1933)
  line L14 (-35.0044, -31.1933) -> (-29.9244, -31.1933)
  line L15 (-29.9244, -31.1933) -> (-29.9244, -36.2733)
  line L16 (-29.9244, -36.2733) -> (-35.0044, -36.2733)
  line L17 (-35.0044, -36.2733) -> (-35.0044, -31.1933)
  line L18 (-48.3394, -78.5039) -> (-46.4344, -78.5039)
  line L19 (-46.4344, -78.5039) -> (-46.4344, -83.5839)
  line L20 (-46.4344, -83.5839) -> (-48.3394, -83.5839)
  line L21 (-48.3394, -83.5839) -> (-48.3394, -78.5039)
  line L22 (-33.0994, -78.5039) -> (-35.0044, -78.5039)
  line L23 (-35.0044, -78.5039) -> (-35.0044, -83.5839)
  line L24 (-35.0044, -83.5839) -> (-33.0994, -83.5839)
  line L25 (-33.0994, -83.5839) -> (-33.0994, -78.5039)
  line L26 (-46.4344, -78.5039) -> (-51.5144, -78.5039)
  line L27 (-51.5144, -78.5039) -> (-51.5144, -83.5839)
  line L28 (-51.5144, -83.5839) -> (-46.4344, -83.5839)
  line L29 (-46.4344, -83.5839) -> (-46.4344, -78.5039)
  line L30 (-35.0044, -78.5039) -> (-29.9244, -78.5039)
  line L31 (-29.9244, -78.5039) -> (-29.9244, -83.5839)
  line L32 (-29.9244, -83.5839) -> (-35.0044, -83.5839)
  line L33 (-35.0044, -83.5839) -> (-35.0044, -78.5039)
  point P0 (0, 0)
  dimension "d166" = 5.08
  dimension "d167" = 5.08
  dimension "d168" = 5.08
  dimension "d169" = 1.905
  dimension "d170" = 1.905
  dimension "d171" = 1.905
  dimension "d172" = 1.905
  dimension "d173" = 5.08
  dimension "d174" = 5.08
  dimension "d175" = 5.08
  dimension "d176" = 5.08
  constraints: 64 end point, 16 parallel, 10 point on line, 8 horizontal, 8 perpendicular
  measures "d166" distance of L1.end L2.end
  measures "d167" distance of L12.end L11.end
  measures "d168" distance of L15.end L16.end
  measures "d169" distance of L1.start L1.end
  measures "d170" distance of L8.end L7.end
  measures "d171" distance of L18.start L18.end
  measures "d172" distance of L22.start L22.end
  measures "d173" distance of L22.end L23.end
  measures "d174" distance of L18.end L19.end
  measures "d175" distance of L28.end L27.end
  measures "d176" distance of L31.end L32.end
extrude "Extrusion16" add sketch "Sketch13" along normal blind 1.905
fillet "Fillet2" radius 3.175 4 edges at (-29.9244, 33.655, -81.0439) (-51.5144, 33.655, -81.0439) (-29.9244, 33.655, -33.7333) (-51.5144, 33.655, -33.7333)
sketch "Sketch14" plane through (-46.4344, 35.56, -36.2733) normal (0, 0, -1) x (-1, 0, 0)
  line L0 (1.905, 0) -> (0, 0) projected
  line L1 (0, 0) -> (0, -1.905) projected
  line L2 (1.905, 0) -> (0, 0)
  line L3 (0, 0) -> (0, -0.9525)
  line L4 (0, -0.9525) -> (1.905, -0.9525)
  line L5 (1.905, -0.9525) -> (1.905, 0)
  line L6 (-11.43, 0) -> (-13.335, 0) projected
  line L7 (-13.335, 0) -> (-11.43, 0)
  line L8 (-11.43, 0) -> (-11.43, -0.9525)
  line L9 (-11.43, -0.9525) -> (-13.335, -0.9525)
  line L10 (-13.335, -0.9525) -> (-13.335, 0)
  point P0 (-46.4344, -35.56)
  point P1 (-11.43, 0)
  dimension "d180" = 0.9525
  dimension "d181" = 0.9525
  constraints: 16 end point, 4 parallel, 2 horizontal, 2 midpoint, 2 perpendicular, 1 point on line
  measures "d180" distance of L0.end point (0, -0.953)
  measures "d181" distance of L7.end L8.end
extrude "Extrusion17" cut sketch "Sketch14" along normal blind 50.8 and the other way blind 12.7
sketch "Sketch15" plane through (0, 38.1, 0) normal (0, 1, 0) x (1, 0, 0)
  line L0 (-29.4242, 96.2295) -> (-14.2582, 96.2295)
  line L1 (-14.2582, 96.2295) -> (-14.2582, 81.5975)
  line L2 (-14.2582, 81.5975) -> (-29.4242, 81.5975)
  line L3 (-29.4242, 81.5975) -> (-29.4242, 96.2295)
  line L4 (-199.3478, 132.7561) -> (16.3943, 132.7561)
  line L5 (16.3943, 132.7561) -> (16.3943, -7.6898)
  line L6 (16.3943, -7.6898) -> (-199.3478, -7.6898)
  line L7 (-199.3478, -7.6898) -> (-199.3478, 132.7561)
  point P0 (0, 0)
  constraints: 16 end point, 4 parallel, 2 horizontal, 2 perpendicular
extrude "Extrusion18" cut sketch "Sketch15" against normal blind 127
body "Solid1"
